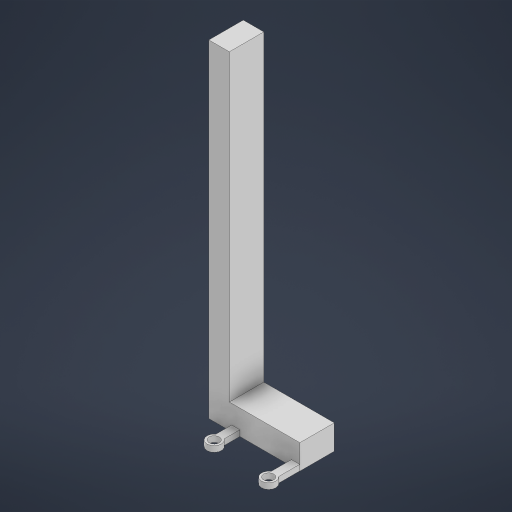
# Autodesk Inventor part: optrode_holder_maelle
Saved by Autodesk Inventor 2023 (Build 270158000, 158)
## iProperties
Created: 2022-10-10
Part Number: optrode_holder_maelle
Material: Generic
Document SubType Name: Modeling
Designer: c4team_RTX3070
Density: 1 g/cm^3
Appearance: Default
Author: c4team_RTX3070
Autodesk Inventor part; units mm, degrees
ref_plane "YZ Plane" through (0, 0, 0) normal (1, 0, 0) x (0, 1, 0)
ref_plane "XZ Plane" through (0, 0, 0) normal (0, 1, 0) x (-1, 0, 0)
ref_plane "XY Plane" through (0, 0, 0) normal (0, 0, 1) x (1, 0, 0)
sketch "Sketch1" plane through (0, 0, 0) normal (0, 1, 0) x (-1, 0, 0)
  line L0 (-0.537, 0.033) -> (-0.537, -0.967)
  line L1 (-0.537, -0.467) -> (-0.537, -2.567)
  line L2 (-0.537, -2.567) -> (10.563, -2.567)
  line L3 (-0.537, -0.967) -> (-0.537, 0.033)
  line L4 (-0.537, 1.633) -> (10.563, 1.633)
  line L5 (-0.537, -0.467) -> (-0.537, 1.633)
  line L6 (10.563, 1.633) -> (10.563, -2.567)
  line L7 (10.563, 1.633) -> (8.063, 1.633)
  line L8 (8.063, 1.633) -> (8.063, -2.567)
  line L9 (10.563, -2.567) -> (10.563, 1.633)
  line L10 (7.7848, 1.633) -> (6.7848, 1.633)
  line L11 (6.7848, 1.633) -> (6.7848, 3.5399)
  line L12 (6.7848, 3.633) -> (7.2848, 3.633)
  line L13 (7.7848, 3.5399) -> (7.7848, 1.633)
  line L14 (0.4848, 1.633) -> (-0.5152, 1.633)
  line L15 (-0.5152, 1.633) -> (-0.5152, 4.1811)
  line L16 (-0.5152, 4.233) -> (0.0393, 4.233)
  line L17 (0.4848, 4.1049) -> (0.4848, 1.633)
  circle A0 centre (7.2848, 4.258) radius 0.625
  arc A1 (7.7848, 3.5399) -> (6.7848, 3.5399) centre (7.2848, 4.258) ccw
  circle A2 centre (0.0393, 4.858) radius 0.625
  arc A3 (0.4848, 4.1049) -> (-0.5152, 4.1811) centre (0.0393, 4.858) ccw
  point P0 (1.1114, -1.7636)
  point P1 (1.1114, -2.7636)
  point P2 (-0.0152, 4.233)
  point P3 (0.0393, 4.0356)
  point P4 (6.7848, 1.633)
  point P5 (-0.5152, 1.633)
  point P6 (7.2848, 1.633)
  dimension "d13" = 1.25
  dimension "d15" = 1.25
  dimension "d4" = 11.1
  dimension "d5" = 4.2
  dimension "d6" = 2.5
  dimension "d9" = 7.3
  dimension "d11" = 1
  dimension "d12" = 1
  dimension "d14" = 1.75
  dimension "d16" = 1.75
  dimension "d17" = 0.6
  dimension "d26" = 2
  constraints: 36 end point, 5 point on line, 4 collinear, 4 horizontal, 4 parallel, 4 point on circle, 3 perpendicular, 2 centre point, 2 vertical, 2 vertical alignment, 1 midpoint, 6 other
  measures "d4" distance of L2.end L1.end
  measures "d5" distance of L4.end L2.end
  measures "d6" distance of L4.end L7.end
  measures "d9" horizontal distance of L12.end point (-0.015, 4.233)
  measures "d11" distance between parallel lines of L11 L13
  measures "d12" distance between parallel lines of L15 L17
  measures "d14" diameter of A1
  measures "d16" diameter of A3
  measures "d17" vertical distance of L12.end point (-0.015, 4.233)
  measures "d26" distance of point (7.285, 1.633) L12.end
extrude "Extrusion1" add sketch "Sketch1" along normal blind 0.7 contours L11 A1 L13 L4
extrude "Extrusion2" add sketch "Sketch1" along normal blind 40 contours L8 L4 L6 L2
extrude "Extrusion3" add sketch "Sketch1" along normal blind 3 contours L5 L4 L8 L2 L1 L0
extrude "Extrusion4" add sketch "Sketch1" along normal blind 0.7 contours L15 A3 L17 L4
body "Solid1"
